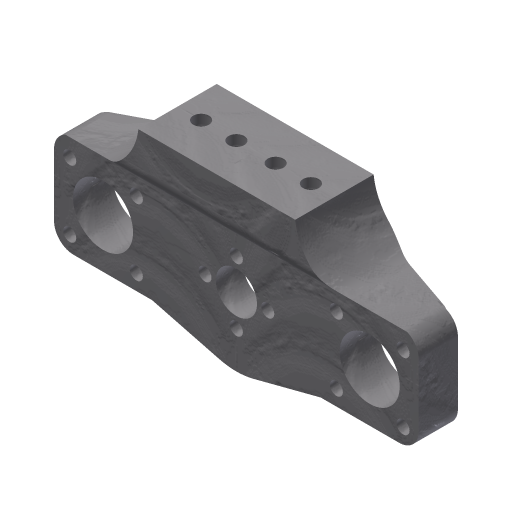
# Autodesk Inventor part: PARA_TUERCA
Saved by Autodesk Inventor 2024 (Build 280153000, 153)
## iProperties
Created: 2024-08-24
Part Number: PARA_TUERCA
Material: Steel, Mild, Welded
Document SubType Name: Modeling
Designer: Niler
Density: 7.85 g/cm^3
Appearance: Weld - Steel Mild
Author: Niler
Autodesk Inventor part; units mm, degrees
ref_plane "YZ Plane" through (0, 0, 0) normal (1, 0, 0) x (0, 1, 0)
ref_plane "XZ Plane" through (0, 0, 0) normal (0, 1, 0) x (-1, 0, 0)
ref_plane "XY Plane" through (0, 0, 0) normal (0, 0, 1) x (1, 0, 0)
sketch "Sketch1" plane through (0, 0, 0) normal (0, 0, 1) x (1, 0, 0)
  line L0 (-20, -5) -> (20, -5)
  line L1 (20, -5) -> (20, 5)
  line L2 (20, 5) -> (-20, 5)
  line L3 (-20, 5) -> (-20, -5)
  line L4 (-20, -5) -> (20, 5) construction
  line L5 (20, -5) -> (-20, 5) construction
  circle A0 centre (0, -18) radius 11.15
  circle A1 centre (0, -18) radius 5.25
  circle A2 centre (0, -18) radius 17.5
  line L6 (-20, -5) -> (-17.2455, -20.9738)
  line L7 (20, -5) -> (17.2455, -20.9738)
  circle A3 centre (0, -10) radius 1.65
  circle A4 centre (-8, -18) radius 1.65
  circle A5 centre (0, -26) radius 1.65
  circle A6 centre (8, -18) radius 1.65
  circle A7 centre (34, -18) radius 7.65
  line L8 (21.5, -30.5) -> (46.5, -30.5)
  line L9 (46.5, -30.5) -> (46.5, -5.5)
  line L10 (46.5, -5.5) -> (21.5, -5.5)
  line L11 (21.5, -5.5) -> (21.5, -30.5)
  line L12 (21.5, -30.5) -> (46.5, -5.5) construction
  line L13 (46.5, -30.5) -> (21.5, -5.5) construction
  circle A8 centre (25.5, -9.5) radius 1.65
  circle A9 centre (42.5, -9.5) radius 1.65
  circle A10 centre (42.5, -26.5) radius 1.65
  circle A11 centre (25.5, -26.5) radius 1.65
  line L14 (46.5, -5.5) -> (20, 0)
  line L15 (21.5, -30.5) -> (4.396, -34.9389)
  line L16 (0, 5) -> (0, 15.3431)
  circle A12 centre (-34, -18) radius 7.65
  line L17 (-21.5, -30.5) -> (-46.5, -30.5)
  line L18 (-46.5, -30.5) -> (-46.5, -5.5)
  line L19 (-46.5, -5.5) -> (-21.5, -5.5)
  line L20 (-21.5, -5.5) -> (-21.5, -30.5)
  line L21 (-21.5, -30.5) -> (-46.5, -5.5) construction
  line L22 (-46.5, -30.5) -> (-21.5, -5.5) construction
  circle A13 centre (-25.5, -9.5) radius 1.65
  circle A14 centre (-42.5, -9.5) radius 1.65
  circle A15 centre (-42.5, -26.5) radius 1.65
  circle A16 centre (-25.5, -26.5) radius 1.65
  line L23 (-46.5, -5.5) -> (-20, 0)
  line L24 (-21.5, -30.5) -> (-4.396, -34.9389)
  point P0 (0, 0)
  point P1 (-4.396, -34.9389)
  dimension "d0" = 22.3
  dimension "d1" = 10.5
  dimension "d2" = 35
  dimension "d3" = 3.3
  dimension "d4" = 8
  dimension "d7" = 360
  dimension "d14" = 40
  dimension "d16" = 23
  dimension "d17" = 10
  dimension "d24" = 15.3
  dimension "d25" = 34
  dimension "d27" = 25
  dimension "d28" = 25
  dimension "d29" = 3.3
  dimension "d30" = 17
  constraints: 50 end point, 17 centre point, 11 symmetric about line, 8 point on line, 6 midpoint, 4 parallel, 4 vertical alignment, 3 equal radius, 3 horizontal alignment, 3 point on circle, 3 tangent, 2 coincident, 2 horizontal, 2 perpendicular, 1 vertical, 14 other
  measures "d0" diameter of A0
  measures "d1" diameter of A1
  measures "d2" diameter of A2
  measures "d3" diameter of A3
  measures "d4" distance of A0.centre A3.centre
  measures "d14" distance of L1.end L2.end
  measures "d16" distance from line of A0.centre L2
  measures "d17" distance of L2.end L0.start
  measures "d24" diameter of A7
  measures "d25" distance of A7.centre A1.centre
  measures "d27" distance of L10.end L9.end
  measures "d28" distance of L9.end L8.end
  measures "d29" diameter of A8
  measures "d30" distance of A9.centre A8.centre
extrude "Extrusion1" add sketch "Sketch1" along normal blind 10 contours L3 L2 L1 L0 A2 | L0 A2 L6 | A2 L0 | L0 A2 | L0 L7 A2 | A0
extrude "Extrusion2" cut sketch "Sketch1" along normal blind 3 contours A0
extrude "Extrusion4" add sketch "Sketch1" along normal blind 10 contours L6 A2 L24 L20 L19 L23 L3 | L19 L20 L17 L18 | L1 L14 L10 L11 L15 A2 L7 | L11 L10 L9 L8
fillet "Fillet1" radius 5 4 edges at (-46.5, -5.5, 5) (-46.5, -30.5, 5) (46.5, -30.5, 5) (46.5, -5.5, 5)
sketch "Sketch4" plane through (-20, 5, 0) normal (0, 1, 0) x (1, 0, 0)
  line L0 (40, 0) -> (0, 0) projected
  line L1 (0, 0) -> (0, -10) projected
  line L2 (40, -10) -> (0, -10) projected
  line L3 (40, 0) -> (40, -10) projected
  point P0 (20, 0)
extrude "Extrusion5" add sketch "Sketch4" along normal blind 5.5
sketch "Sketch5" plane through (-20, 10.5, 0) normal (0, 1, 0) x (1, 0, 0)
  line L0 (40, 0) -> (0, 0) projected
  line L1 (0, 0) -> (0, -10) projected
  line L2 (0, -10) -> (40, -10) projected
  line L3 (40, -10) -> (40, 0) projected
  line L4 (40, 0) -> (0, -10)
  line L5 (0, 5) -> (40, 5)
  line L6 (40, 5) -> (40, -15)
  line L7 (40, -15) -> (0, -15)
  line L8 (0, -15) -> (0, 5)
  line L9 (0, 5) -> (40, -15) construction
  line L10 (40, 5) -> (0, -15) construction
  point P0 (20, 0)
  point P1 (20, -5)
  constraints: 14 end point, 3 midpoint, 2 parallel, 1 horizontal, 1 perpendicular
extrude "Extrusion6" add sketch "Sketch5" against normal blind 10.5
chamfer "Chamfer1" distance 5 angle 45 2 edges at (0, 0, 10) (0, 0, 0)
sketch "Sketch7" plane through (-20, 10.5, 0) normal (0, 1, 0) x (1, 0, 0)
  line L0 (0, 5) -> (0, -15) projected
  line L1 (0, -15) -> (40, -15) projected
  line L2 (40, -15) -> (40, 5) projected
  line L3 (40, 5) -> (0, 5) projected
  line L4 (0, -5) -> (40, -5)
  line L5 (20, -5) -> (34, -5)
  line L6 (34, -5) -> (25, -5)
  circle A0 centre (34, -5) radius 2
  line L7 (34, -5) -> (25, -5)
  circle A1 centre (25, -5) radius 2
  line L8 (20, -5) -> (20, -8)
  circle A2 centre (6, -5) radius 2
  circle A3 centre (15, -5) radius 2
  point P0 (20, 0)
  dimension "d45" = 14
  dimension "d47" = 4
  dimension "d48" = 9
  dimension "d49" = 4
  constraints: 10 end point, 4 centre point, 3 midpoint, 2 coincident, 2 point on line, 2 symmetric about line, 1 horizontal, 1 vertical, 2 other
  measures "d45" distance of L5.start L5.end
  measures "d47" diameter of A0
  measures "d48" distance of L7.start L6.end
  measures "d49" diameter of A1
fillet "Fillet2" radius 15 2 edges at (-20, 0, 5) (20, 0, 5)
fillet "Fillet3" radius 5 2 edges at (0, 0, -5) (0, 0, 15)
extrude "Extrusion7" cut sketch "Sketch7" against normal blind 18 contours A2 L4 | L4 A2 | A0 L4 | L4 A0 | A3 L4 | L4 A3 | A1 L4 | L4 A1
body "Solid1"
